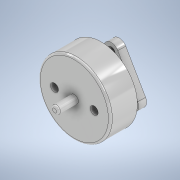
# Autodesk Inventor part: Motor_18mm
Saved by Autodesk Inventor 2021 (Build 250183000, 183)
## iProperties
Created: 2024-05-10
Part Number: Motor_18mm
Material: Generic
Document SubType Name: Modeling
Designer: Lukas
Density: 1 g/cm^3
Appearance: Default
Author: Lukas
Autodesk Inventor part; units mm, degrees
ref_plane "YZ Plane" through (0, 0, 0) normal (1, 0, 0) x (0, 1, 0)
ref_plane "XZ Plane" through (0, 0, 0) normal (0, 1, 0) x (-1, 0, 0)
ref_plane "XY Plane" through (0, 0, 0) normal (0, 0, 1) x (1, 0, 0)
sketch "Sketch1" plane through (0, 0, 0) normal (0, 0, 1) x (1, 0, 0)
  circle A0 centre (0, 0) radius 9.075
  dimension "d0" = 18.15
  constraints: 1 centre point, 1 coincident
  measures "d0" diameter of A0
extrude "Extrusion1" add sketch "Sketch1" along normal blind 6.8
sketch "Sketch6" plane through (0, 0, 6.8) normal (0, 0, 1) x (1, 0, 0)
  circle A0 centre (-5, 0) radius 1
  circle A1 centre (5, 0) radius 1
  point P0 (0, 0)
  dimension "d25" = 5
  dimension "d26" = 5
  dimension "d27" = 2
  constraints: 2 centre point, 2 horizontal alignment, 1 equal radius
  measures "d25" distance of point (0, 0) A0.centre
  measures "d26" distance of A1.centre point (0, 0)
  measures "d27" diameter of A0
extrude "Extrusion6" cut sketch "Sketch6" against normal blind 1.6
sketch "Sketch2" plane through (0, 0, 6.8) normal (0, 0, 1) x (1, 0, 0)
  circle A0 centre (0, 0) radius 1
  dimension "d3" = 2
  constraints: 1 centre point, 1 coincident
  measures "d3" diameter of A0
extrude "Extrusion2" add sketch "Sketch2" along normal blind 5
sketch "Sketch3" plane through (0, 0, 0) normal (0, 0, -1) x (-1, 0, 0)
  circle A0 centre (0, 0) radius 3.5
  dimension "d6" = 7
  constraints: 1 centre point, 1 coincident
  measures "d6" diameter of A0
extrude "Extrusion3" add sketch "Sketch3" along normal blind 2.5
sketch "Sketch4" plane through (0, 0, -2.5) normal (0, 0, -1) x (-1, 0, 0)
  circle A0 centre (0, 5.7735) radius 1
  circle A1 centre (-5, -2.8868) radius 1
  circle A2 centre (5, -2.8868) radius 1
  arc A3 (1.6627, 6.7334) -> (-1.6627, 6.7334) centre (0, 5.7735) ccw
  arc A4 (5, -4.8066) -> (6.6627, -1.9268) centre (5, -2.8868) ccw
  arc A5 (-6.6627, -1.9268) -> (-5, -4.8066) centre (-5, -2.8868) ccw
  line L0 (-6.6627, -1.9268) -> (-1.6627, 6.7334)
  line L1 (1.6627, 6.7334) -> (6.6627, -1.9268)
  line L2 (5, -4.8066) -> (-5, -4.8066)
  point P0 (0, 0)
  dimension "d9" = 10
  dimension "d10" = 10
  dimension "d11" = 10
  dimension "d12" = 5
  dimension "d13" = 2
  dimension "d17" = 5.7735
  dimension "d18" = 5.7735
  dimension "d19" = 12.5
  constraints: 6 centre point, 6 end point, 6 point on circle, 6 tangent, 4 equal radius, 3 coincident, 1 vertical alignment
  measures "d9" distance of A1.centre A0.centre
  measures "d10" distance of A2.centre A0.centre
  measures "d11" distance of A2.centre A1.centre
  measures "d12" horizontal distance of point (0, 0) A1.centre
  measures "d13" diameter of A0
  measures "d17" distance of A0.centre point (0, 0)
  measures "d18" distance of A1.centre point (0, 0)
extrude "Extrusion4" add sketch "Sketch4" along normal blind 2
sketch "Sketch5" plane through (0, 0, -4.5) normal (0, 0, -1) x (-1, 0, 0)
  circle A0 centre (0, 0) radius 2.15
  dimension "d22" = 4.3
  constraints: 1 centre point, 1 coincident
  measures "d22" diameter of A0
extrude "Extrusion5" add sketch "Sketch5" along normal blind 1.6
fillet "Fillet1" radius 0.5 2 edges at (-1, 0, 11.8) (-9.075, 0, 6.8)
chamfer "Chamfer1" distance 1 angle 45 1 edges at (2.15, 0, -6.1)
equation "\"d26\" = d25"
equation "\"d10\" = d9"
equation "\"d11\" = d9"
equation "\"d12\" = 0.5 * d11"
equation "\"d17\" = d18"
body "Solid1"
